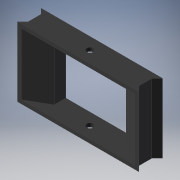
# Autodesk Inventor part: Part3
Saved by Autodesk Inventor 2019 (Build 230136000, 136)
## iProperties
Created: 2020-01-30
Part Number: Part3
Material: Generic
Document SubType Name: Modeling
Designer: marsikovabarbora
Density: 1 g/cm^3
Appearance: Default
Author: marsikovabarbora
Autodesk Inventor part; units mm, degrees
ref_plane "YZ Plane" through (0, 0, 0) normal (1, 0, 0) x (0, 1, 0)
ref_plane "XZ Plane" through (0, 0, 0) normal (0, 1, 0) x (-1, 0, 0)
ref_plane "XY Plane" through (0, 0, 0) normal (0, 0, 1) x (1, 0, 0)
sketch "Sketch1" plane through (0, 0, 0) normal (0, 1, 0) x (-1, 0, 0)
  line L0 (41.2832, 0) -> (-41.2832, 0) construction
  line L1 (0, -8.0192) -> (0, 8.0192) construction
  line L2 (26.9, 0) -> (26.9, -3.14)
  line L3 (26.9, -3.14) -> (29.488, -5.728)
  line L4 (29.488, -5.728) -> (0, -5.728)
  line L5 (26.9, 0) -> (26.9, 3.14)
  line L6 (26.9, 3.14) -> (29.488, 5.728)
  line L7 (29.488, 5.728) -> (0, 5.728)
  line L8 (-26.9, 0) -> (-26.9, -3.14)
  line L9 (-26.9, -3.14) -> (-29.488, -5.728)
  line L10 (-29.488, -5.728) -> (0, -5.728)
  line L11 (-26.9, 0) -> (-26.9, 3.14)
  line L12 (-26.9, 3.14) -> (-29.488, 5.728)
  line L13 (-29.488, 5.728) -> (0, 5.728)
  point P0 (0, 0)
  dimension "d0" = 26.9
  dimension "d1" = 3.14
  dimension "d2" = 3.66
  dimension "d3" = 135
  constraints: 24 end point, 8 symmetric about line, 2 point on line, 1 perpendicular, 1 vertical
  measures "d0" distance between parallel lines of L1 L2
  measures "d1" distance of L2.start L2.end
  measures "d2" distance of L2.end L3.end
  measures "d3" angle of L2 L3
extrude "Extrusion1" add sketch "Sketch1" along normal blind 33.5
sketch "Sketch2" plane through (-29.488, 0, 5.728) normal (0, 0, 1) x (1, 0, 0)
  line L0 (58.976, 0) -> (0, 0) construction
  line L1 (58.976, 0) -> (58.976, 33.5) construction
  line L2 (0, 33.5) -> (58.976, 33.5) construction
  line L3 (0, 0) -> (0, 33.5) construction
  line L4 (29.488, -6.8) -> (29.488, 40.8) construction
  line L5 (46.988, 1.75) -> (11.988, 1.75)
  line L6 (11.988, 1.75) -> (11.988, 31.75)
  line L7 (11.988, 31.75) -> (46.988, 31.75)
  line L8 (46.988, 31.75) -> (46.988, 1.75)
  line L9 (46.988, 1.75) -> (11.988, 31.75) construction
  line L10 (11.988, 1.75) -> (46.988, 31.75) construction
  point P0 (29.488, 16.75)
  dimension "d16" = 30
  dimension "d17" = 35
  dimension "d18" = 16.75
  constraints: 12 end point, 2 midpoint, 2 parallel, 1 horizontal, 1 perpendicular, 1 point on line
  measures "d16" distance of L7.end L5.start
  measures "d17" distance of L6.end L7.end
  measures "d18" distance from line of L0 point (29.488, 16.75)
extrude "Extrusion2" cut sketch "Sketch2" against normal through all
sketch "Sketch3" plane through (0, 33.5, 0) normal (0, 1, 0) x (1, 0, 0)
  line L0 (-26.9, 3.14) -> (-26.9, -3.14) construction
  line L1 (-26.9, -3.14) -> (-29.488, -5.728) construction
  line L2 (-29.488, -5.728) -> (29.488, -5.728) construction
  line L3 (29.488, -5.728) -> (26.9, -3.14) construction
  line L4 (26.9, -3.14) -> (26.9, 3.14) construction
  line L5 (26.9, 3.14) -> (29.488, 5.728) construction
  line L6 (29.488, 5.728) -> (-29.488, 5.728) construction
  line L7 (-29.488, 5.728) -> (-26.9, 3.14) construction
  circle A0 centre (0, 0) radius 1.7
  dimension "d10" = 3.4
  constraints: 1 centre point, 1 coincident
  measures "d10" diameter of A0
extrude "Extrusion3" cut sketch "Sketch3" against normal through all
ref_plane "Work Plane1" through (0, 29.5, 5.728) normal (0, -1, 0) x (1, 0, 0)
sketch "Sketch4" plane through (0, 29.5, 5.728) normal (0, -1, 0) x (1, 0, 0)
  circle A0 centre (0, -5.728) radius 1.7 construction
  line L0 (-26.9, -8.868) -> (-26.9, -2.588) construction
  line L1 (-26.9, -2.588) -> (-29.488, 0) construction
  line L2 (-29.488, 0) -> (29.488, 0) construction
  line L3 (29.488, 0) -> (26.9, -2.588) construction
  line L4 (26.9, -2.588) -> (26.9, -8.868) construction
  line L5 (26.9, -8.868) -> (29.488, -11.456) construction
  line L6 (29.488, -11.456) -> (-29.488, -11.456) construction
  line L7 (-29.488, -11.456) -> (-26.9, -8.868) construction
  line L8 (12.5, 0) -> (12.5, -11.456) construction
  line L9 (-12.5, 0) -> (-12.5, -11.456) construction
  line L10 (0, -5.728) -> (21.3772, 0)
  line L11 (0, -5.728) -> (22.1313, -5.728) construction
  line L12 (0, -13.7472) -> (0, 2.2912) construction
  line L13 (0, -5.728) -> (-21.3772, 0)
  line L14 (-21.3772, 0) -> (21.3772, 0)
  line L15 (29.488, 0) -> (-29.488, 0) construction
  dimension "d13" = 15
  constraints: 8 end point, 1 collinear, 1 equal length, 1 horizontal, 1 point on line, 1 symmetric about line
  measures "d13" angle of L11 L10
extrude "Extrusion4" [suppressed]
chamfer "Chamfer1" distance 10 angle 30 2 edges at (-17.5, 16.75, 5.728) (17.5, 16.75, 5.728) measured on face at (25.492, 11.75, 5.728)
equation "\"d18\" = 0.5 * d4"
equation "\"d4\" = 33.5"
body "Solid1"
